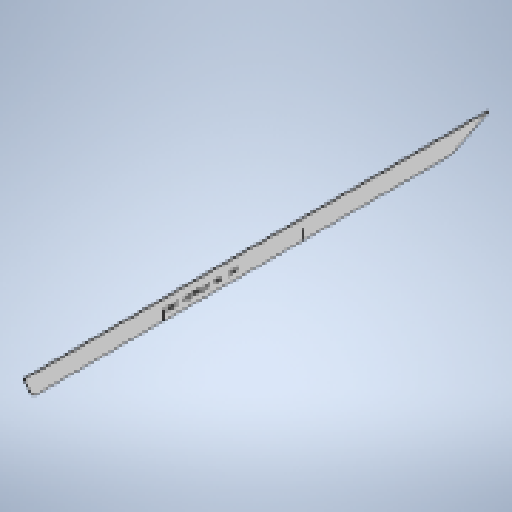
# Autodesk Inventor part: MSC 110 STRINGER CONE
Saved by Autodesk Inventor 2025 (Build 290162010, 162A)
## iProperties
Created: 2024-06-26
Part Number: MSC 110 STRINGER CONE
Material: Stainless Steel
Document SubType Name: Sheet Metal
Designer: pokla
Density: 8 g/cm^3
Sheet Metal Rule: AISI304 3mm Die 32
Appearance: Default
Stock Number: МОО 110 стрингер конус
Mass: 1037.19 g
Surface Area: 923.652 cm^2
Volume: 129.648 cm^3
Flat Pattern Width: 5 cm
Flat Pattern Length: 121.598 cm
Flat Pattern Area: 607.988 cm^2
Sheet Metal Width: 50,000 mm
Sheet Metal Length: 1215,975 mm
Sheet Metal Area: 60798,754 mm^2
Author: pokla
Autodesk Inventor part; units mm, degrees
ref_plane "YZ Plane" through (0, 0, 0) normal (1, 0, 0) x (0, 1, 0)
ref_plane "XZ Plane" through (0, 0, 0) normal (0, 1, 0) x (-1, 0, 0)
ref_plane "XY Plane" through (0, 0, 0) normal (0, 0, 1) x (1, 0, 0)
sketch "Sketch2" plane through (0, 0, 0) normal (1, 0, 0) x (0, 1, 0)
  line L0 (0, 0) -> (1220, 0)
  line L1 (1220, 0) -> (1220, -50)
  line L2 (1220, -50) -> (0, -50)
  line L3 (0, -50) -> (0, 0)
  line L4 (1220, -50) -> (1183.2713, 0) construction
  line L5 (1220, 0) -> (1120, -50)
  line L6 (0, 0) -> (25, -50)
  dimension "d28" = 1220
  dimension "d29" = 50
  dimension "d31" = 36.3
  dimension "d32" = 63.435
  dimension "d36" = 63.435
  measures "d28" distance of L1.end L2.end
  measures "d29" distance of L0.end L1.end
  measures "d31" angle of L1 L4
  measures "d32" angle of L5 L1
  measures "d36" angle of L0 L6
extrude "Plate2" add sketch "Sketch2" along normal blind 3 contours L0 L5 L2 L6
chamfer "Corner Chamfer1" distance 3 angle 45 2 edges at (1.5, 1220, 0) (1.5, 0, 0)
fillet "Corner Round1" radius 6 2 edges at (1.5, 25, -50) (1.5, 1120, -50)
sketch "Sketch3" plane through (3, 0, 0) normal (1, 0, 0) x (0, 0, -1)
  line L0 (24, 364.5) -> (50, 364.5)
  line L1 (50, 364.5) -> (50, 367.5)
  line L2 (50, 367.5) -> (24, 367.5)
  line L3 (24, 367.5) -> (24, 364.5)
  line L4 (50, 1118.5836) -> (50, 28.7082) projected
  line L5 (50, 366) -> (0, 366) construction
  line L6 (0, 3) -> (0, 1217) projected
  line L7 (50, 732) -> (0, 732) construction
  line L8 (24, 730.5) -> (50, 730.5)
  line L9 (50, 730.5) -> (50, 733.5)
  line L10 (50, 733.5) -> (24, 733.5)
  line L11 (24, 733.5) -> (24, 730.5)
  point P0 (0, 0)
  point P1 (50, 730.5)
  point P2 (50, 733.5)
  dimension "d39" = 26
  dimension "d40" = 3
  dimension "d41" = 366
  dimension "d42" = 732
  dimension "d43" = 3
  dimension "d44" = 26
  constraints: 20 end point, 4 parallel, 4 point on line, 3 horizontal, 3 perpendicular, 2 midpoint
  measures "d39" distance of L2.end L1.end
  measures "d40" distance of L0.end L1.end
  measures "d41" distance from line of point (0, 0) L5
  measures "d42" distance from line of point (0, 0) L7
  measures "d43" distance of L8.end L9.end
  measures "d44" distance of L9.end L10.end
extrude "Extrusion1" cut sketch "Sketch3" against normal through all
sketch "Sketch4" plane through (3, 0, 0) normal (1, 0, 0) x (0, 0, -1)
  line L0 (13.0577, 558.8324) -> (33.8114, 558.8324) construction
  line L1 (33.8114, 558.8324) -> (33.8114, 335.0608) construction
  line L2 (33.8114, 335.0608) -> (13.0577, 335.0608) construction
  line L3 (13.0577, 335.0608) -> (13.0577, 558.8324) construction
  point P0 (0, 0)
  constraints: 2 other
mark "Mark1"
equation "\"d41\" = 0.3 * Конус_длина_борт"
equation "\"d42\" = 0.6 * Конус_длина_борт"
equation "\"d28\" = Конус_длина_борт"
equation "\"d32\" = Конус_Угол_борт"
equation "\"d36\" = Конус_Угол_борт"
equation "\"d40\" = Thickness"
equation "\"d43\" = Thickness"
equation "\"d44\" = d39"
equation "\"d30\" = Thickness"
equation "\"BendReliefWidth\" = Thickness"
equation "\"BendReliefDepth\" = 0.5 * Thickness"
equation "\"CornerReliefSize\" = 4 * Thickness"
equation "\"MinimumRemnant\" = 2 * Thickness"
equation "\"TransitionRadius\" = BendRadius"
equation "\"JacobiRadiusSize\" = BendRadius"
equation "\"GapSize\" = Thickness"
equation "\"Конус_длина_борт\" = 1220"
equation "\"Конус_Угол_борт\" = 63.434949deg"
equation "\"Thickness\" = 3"
equation "\"BendRadius\" = 5"
body "Solid2"
